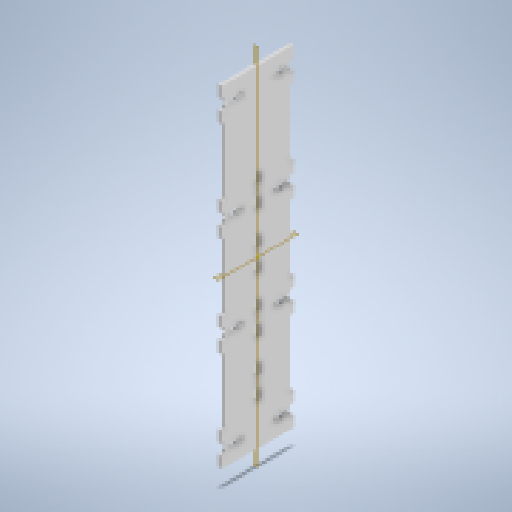
# Autodesk Inventor part: Крепление для крепления механизма головы
Saved by Autodesk Inventor 2023.2 (Build 272271030, 271C)
## iProperties
Created: 2024-02-18
Part Number: Крепление для крепления механизма головы
Material: Типовые
Document SubType Name: Modeling
Designer: I9232
Density: 1 g/cm^3
Appearance: Серо-синий
Mass: 21.1298 g
Surface Area: 152.682 cm^2
Volume: 21.1298 cm^3
Author: I9232
Autodesk Inventor part; units mm, degrees
ref_plane "YZ Plane" through (0, 0, 0) normal (1, 0, 0) x (0, 1, 0)
sketch "Эскиз1" plane through (0, 0, 0) normal (1, 0, 0) x (0, 1, 0)
  line L0 (-150, 29.5) -> (150, 29.5)
  line L1 (150, 29.5) -> (150, -29.5)
  line L2 (150, -29.5) -> (-150, -29.5)
  line L3 (-150, -29.5) -> (-150, 29.5)
  line L4 (-150, 29.5) -> (150, -29.5) construction
  line L5 (150, 29.5) -> (-150, -29.5) construction
  point P0 (0, 0)
  dimension "d0" = 300
  dimension "d1" = 59
  constraints: 12 end point, 2 midpoint, 2 parallel, 1 horizontal, 1 perpendicular
  measures "d0" distance of L0.start L0.end
  measures "d1" distance of L0.end L1.end
extrude "Выдавливание1" add sketch "Эскиз1" along normal mid plane 3
sketch "Эскиз2" plane through (0, 0, 0) normal (1, 0, 0) x (0, 1, 0)
  point P0 (0, 0)
sketch "Эскиз4" plane through (1.5, -150, -29.5) normal (0, 0, -1) x (-1, 0, 0)
  line L0 (3, 0) -> (0, 0)
  line L1 (0, 0) -> (0, 10)
  line L2 (0, 10) -> (3, 10)
  line L3 (3, 10) -> (3, 0)
  line L4 (3, 0) -> (3, 300) projected
  line L5 (0, 0) -> (0, 300) projected
  line L6 (3, 20) -> (0, 20)
  line L7 (0, 20) -> (0, 30)
  line L8 (0, 30) -> (3, 30)
  line L9 (3, 30) -> (3, 20)
  line L10 (3, 120) -> (0, 120)
  line L11 (0, 120) -> (0, 110)
  line L12 (0, 110) -> (3, 110)
  line L13 (3, 110) -> (3, 120)
  line L14 (3, 90) -> (3, 100)
  line L15 (3, 100) -> (0, 100)
  line L16 (0, 100) -> (0, 90)
  line L17 (0, 90) -> (3, 90)
  line L18 (3, 150) -> (0, 150) construction
  line L19 (3, 300) -> (0, 300)
  line L20 (0, 300) -> (0, 290)
  line L21 (0, 290) -> (3, 290)
  line L22 (3, 290) -> (3, 300)
  line L23 (3, 280) -> (0, 280)
  line L24 (0, 280) -> (0, 270)
  line L25 (0, 270) -> (3, 270)
  line L26 (3, 270) -> (3, 280)
  line L27 (3, 180) -> (0, 180)
  line L28 (0, 180) -> (0, 190)
  line L29 (0, 190) -> (3, 190)
  line L30 (3, 190) -> (3, 180)
  line L31 (3, 210) -> (3, 200)
  line L32 (3, 200) -> (0, 200)
  line L33 (0, 200) -> (0, 210)
  line L34 (0, 210) -> (3, 210)
  point P0 (1.5, 150)
  point P1 (1.5, 120)
  point P2 (1.5, 100)
  point P3 (1.5, 180)
  point P4 (1.5, 200)
  point P5 (0, 200)
  point P6 (0, 180)
  point P7 (0, 120)
  point P8 (0, 100)
  dimension "d14" = 10
  dimension "d18" = 20
  dimension "d23" = 30
  dimension "d26" = 20
  constraints: 66 end point, 16 symmetric about line, 4 parallel, 3 midpoint, 2 horizontal, 2 perpendicular, 2 point on line, 2 vertical, 1 collinear, 17 other
  measures "d14" distance of L0.end L1.end
  measures "d18" distance of L1.end L7.end
  measures "d23" distance of point (1.5, 120) point (1.5, 150)
  measures "d26" distance of L10.start L14.end
extrude "Выдавливание2" add sketch "Эскиз4" along normal blind 3 contours L0 L1 L2 L3 | L6 L5 L8 L4 | L17 L5 L15 L4 | L12 L5 L10 L4 | L27 L5 L29 L4 | L32 L5 L34 L4 | L25 L5 L23 L4 | L21 L5 L19 L4
sketch "Эскиз5" plane through (1.5, -150, 29.5) normal (0, 0, 1) x (1, 0, 0)
  line L0 (0, 30) -> (0, 20)
  line L1 (0, 20) -> (-3, 20)
  line L2 (-3, 20) -> (-3, 30)
  line L3 (-3, 30) -> (0, 30)
  line L4 (-3, 10) -> (0, 10)
  line L5 (0, 10) -> (0, 0)
  line L6 (0, 0) -> (-3, 0)
  line L7 (-3, 0) -> (-3, 10)
  line L8 (-3, 90) -> (-3, 100)
  line L9 (-3, 100) -> (0, 100)
  line L10 (0, 100) -> (0, 90)
  line L11 (0, 90) -> (-3, 90)
  line L12 (-3, 110) -> (-3, 120)
  line L13 (-3, 120) -> (0, 120)
  line L14 (0, 120) -> (0, 110)
  line L15 (0, 110) -> (-3, 110)
  line L16 (-3, 180) -> (-3, 190)
  line L17 (-3, 190) -> (0, 190)
  line L18 (0, 190) -> (0, 180)
  line L19 (0, 180) -> (-3, 180)
  line L20 (-3, 200) -> (-3, 210)
  line L21 (-3, 210) -> (0, 210)
  line L22 (0, 210) -> (0, 200)
  line L23 (0, 200) -> (-3, 200)
  line L24 (0, 280) -> (0, 270)
  line L25 (0, 270) -> (-3, 270)
  line L26 (-3, 270) -> (-3, 280)
  line L27 (-3, 280) -> (0, 280)
  line L28 (0, 300) -> (0, 290)
  line L29 (0, 290) -> (-3, 290)
  line L30 (-3, 290) -> (-3, 300)
  line L31 (-3, 300) -> (0, 300)
  point P0 (-1.5, 150)
  constraints: 64 end point
extrude "Выдавливание3" add sketch "Эскиз5" along normal blind 3
sketch "Эскиз6" plane through (1.5, 0, 0) normal (1, 0, 0) x (0, 0, -1)
  line L0 (29.5, -130) -> (29.5, -140) projected
  line L1 (13.9, -136.5) -> (13.9, -133.5)
  line L2 (29.5, -133.5) -> (29.5, -136.5)
  line L3 (21.4, -138.05) -> (18.9, -138.05)
  line L4 (18.9, -131.95) -> (21.4, -131.95)
  line L5 (29.5, -136.5) -> (21.4, -136.5)
  line L6 (18.9, -136.5) -> (13.9, -136.5)
  line L7 (21.4, -131.95) -> (21.4, -133.5)
  line L8 (21.4, -136.5) -> (21.4, -138.05)
  line L9 (18.9, -138.05) -> (18.9, -136.5)
  line L10 (18.9, -133.5) -> (18.9, -131.95)
  line L11 (13.9, -133.5) -> (18.9, -133.5)
  line L12 (21.4, -133.5) -> (29.5, -133.5)
  line L13 (21.4, -138.05) -> (18.9, -131.95) construction
  line L14 (18.9, -138.05) -> (21.4, -131.95) construction
  line L15 (13.9, -46.51) -> (13.9, -43.51)
  line L16 (29.5, -43.5) -> (29.5, -46.5)
  line L17 (21.4, -48.06) -> (18.9, -48.06)
  line L18 (18.9, -41.96) -> (21.4, -41.96)
  line L19 (29.5, -46.5) -> (21.4, -46.5)
  line L20 (18.9, -46.51) -> (13.9, -46.51)
  line L21 (21.4, -41.96) -> (21.4, -43.5)
  line L22 (21.4, -46.5) -> (21.4, -48.06)
  line L23 (18.9, -48.06) -> (18.9, -46.51)
  line L24 (18.9, -43.51) -> (18.9, -41.96)
  line L25 (13.9, -43.51) -> (18.9, -43.51)
  line L26 (21.4, -43.5) -> (29.5, -43.5)
  line L27 (21.4, -48.06) -> (18.9, -41.96) construction
  line L28 (18.9, -48.06) -> (21.4, -41.96) construction
  line L29 (29.5, -50) -> (29.5, -40) projected
  line L30 (0, -102.6029) -> (0, -84.657) construction
  line L31 (-13.9, -136.5) -> (-13.9, -133.5)
  line L32 (-21.4, -138.05) -> (-18.9, -138.05)
  line L33 (-18.9, -131.95) -> (-21.4, -131.95)
  line L34 (-29.5, -136.5) -> (-21.4, -136.5)
  line L35 (-18.9, -136.5) -> (-13.9, -136.5)
  line L36 (-21.4, -131.95) -> (-21.4, -133.5)
  line L37 (-21.4, -136.5) -> (-21.4, -138.05)
  line L38 (-18.9, -138.05) -> (-18.9, -136.5)
  line L39 (-18.9, -133.5) -> (-18.9, -131.95)
  line L40 (-13.9, -133.5) -> (-18.9, -133.5)
  line L41 (-21.4, -133.5) -> (-29.5, -133.5)
  line L42 (-21.4, -138.05) -> (-18.9, -131.95) construction
  line L43 (-18.9, -138.05) -> (-21.4, -131.95) construction
  line L44 (-18.9, -41.96) -> (-21.4, -41.96)
  line L45 (-18.9, -48.06) -> (-21.4, -41.96) construction
  line L46 (-21.4, -48.06) -> (-18.9, -48.06)
  line L47 (-21.4, -48.06) -> (-18.9, -41.96) construction
  line L48 (-21.4, -41.96) -> (-21.4, -43.5)
  line L49 (-21.4, -46.5) -> (-21.4, -48.06)
  line L50 (-29.5, -43.5) -> (-29.5, -46.5)
  line L51 (-21.4, -43.5) -> (-29.5, -43.5)
  line L52 (-29.5, -46.5) -> (-21.4, -46.5)
  line L53 (-18.9, -43.51) -> (-18.9, -41.96)
  line L54 (-18.9, -48.06) -> (-18.9, -46.51)
  line L55 (-18.9, -46.51) -> (-13.9, -46.51)
  line L56 (-13.9, -43.51) -> (-18.9, -43.51)
  line L57 (-13.9, -46.51) -> (-13.9, -43.51)
  line L58 (7.1408, 0) -> (-5.4038, 0) construction
  line L59 (13.9, 136.5) -> (13.9, 133.5)
  line L60 (29.5, 133.5) -> (29.5, 136.5)
  line L61 (21.4, 138.05) -> (18.9, 138.05)
  line L62 (18.9, 131.95) -> (21.4, 131.95)
  line L63 (29.5, 136.5) -> (21.4, 136.5)
  line L64 (18.9, 136.5) -> (13.9, 136.5)
  line L65 (21.4, 131.95) -> (21.4, 133.5)
  line L66 (21.4, 136.5) -> (21.4, 138.05)
  line L67 (18.9, 138.05) -> (18.9, 136.5)
  line L68 (18.9, 133.5) -> (18.9, 131.95)
  line L69 (13.9, 133.5) -> (18.9, 133.5)
  line L70 (21.4, 133.5) -> (29.5, 133.5)
  line L71 (21.4, 138.05) -> (18.9, 131.95) construction
  line L72 (18.9, 138.05) -> (21.4, 131.95) construction
  line L73 (18.9, 41.96) -> (21.4, 41.96)
  line L74 (18.9, 48.06) -> (21.4, 41.96) construction
  line L75 (21.4, 48.06) -> (18.9, 48.06)
  line L76 (21.4, 48.06) -> (18.9, 41.96) construction
  line L77 (21.4, 41.96) -> (21.4, 43.5)
  line L78 (21.4, 46.5) -> (21.4, 48.06)
  line L79 (29.5, 43.5) -> (29.5, 46.5)
  line L80 (21.4, 43.5) -> (29.5, 43.5)
  line L81 (29.5, 46.5) -> (21.4, 46.5)
  line L82 (18.9, 43.51) -> (18.9, 41.96)
  line L83 (18.9, 48.06) -> (18.9, 46.51)
  line L84 (18.9, 46.51) -> (13.9, 46.51)
  line L85 (13.9, 43.51) -> (18.9, 43.51)
  line L86 (13.9, 46.51) -> (13.9, 43.51)
  line L87 (0, 102.6029) -> (0, 84.657) construction
  line L88 (-21.4, 131.95) -> (-21.4, 133.5)
  line L89 (-21.4, 138.05) -> (-18.9, 138.05)
  line L90 (-21.4, 138.05) -> (-18.9, 131.95) construction
  line L91 (-18.9, 138.05) -> (-18.9, 136.5)
  line L92 (-18.9, 131.95) -> (-21.4, 131.95)
  line L93 (-13.9, 133.5) -> (-18.9, 133.5)
  line L94 (-13.9, 136.5) -> (-13.9, 133.5)
  line L95 (-18.9, 136.5) -> (-13.9, 136.5)
  line L96 (-18.9, 138.05) -> (-21.4, 131.95) construction
  line L97 (-18.9, 46.51) -> (-13.9, 46.51)
  line L98 (-13.9, 43.51) -> (-18.9, 43.51)
  line L99 (-13.9, 46.51) -> (-13.9, 43.51)
  line L100 (-18.9, 133.5) -> (-18.9, 131.95)
  line L101 (-21.4, 136.5) -> (-21.4, 138.05)
  line L102 (-21.4, 133.5) -> (-29.5, 133.5)
  line L103 (-29.5, 136.5) -> (-21.4, 136.5)
  line L104 (-18.9, 41.96) -> (-21.4, 41.96)
  line L105 (-18.9, 48.06) -> (-18.9, 46.51)
  line L106 (-21.4, 48.06) -> (-18.9, 48.06)
  line L107 (-21.4, 46.5) -> (-21.4, 48.06)
  line L108 (-18.9, 43.51) -> (-18.9, 41.96)
  line L109 (-18.9, 48.06) -> (-21.4, 41.96) construction
  line L110 (-21.4, 48.06) -> (-18.9, 41.96) construction
  line L111 (-21.4, 41.96) -> (-21.4, 43.5)
  line L112 (-29.5, 46.5) -> (-21.4, 46.5)
  line L113 (-21.4, 43.5) -> (-29.5, 43.5)
  line L114 (-29.5, 129.75) -> (-29.5, 139.75)
  line L115 (-29.5, 43.5) -> (-29.5, 46.5)
  line L116 (-29.5, -136.5) -> (-29.5, -133.5)
  line L117 (-29.5, -140) -> (-29.5, -130) projected
  point P0 (0, 0)
  point P1 (29.5, -135)
  point P2 (21.4, -47.28)
  point P3 (29.5, -45)
  point P4 (-21.4, -47.28)
  point P5 (29.5, 135)
  point P6 (21.4, 47.28)
  point P7 (29.5, 45)
  point P8 (-21.4, 47.28)
  point P9 (29.5, -133.5)
  dimension "d36" = 3
  dimension "d40" = 2.5
  dimension "d42" = 8.1
  dimension "d43" = 8.1
  dimension "d44" = 5
  dimension "d45" = 3
  dimension "d46" = 3
  dimension "d48" = 2.5
  dimension "d51" = 8.1
  dimension "d52" = 5
  dimension "d53" = 3
  dimension "d54" = 8.1
  dimension "d58" = 6.1
  dimension "d59" = 6.1
  constraints: 230 end point, 79 symmetric about line, 20 parallel, 8 perpendicular, 7 horizontal, 5 midpoint, 4 equal length, 2 point on line, 1 collinear, 1 vertical
  measures "d36" distance of L1.start L1.end
  measures "d40" distance of L3.start L3.end
  measures "d42" distance between parallel lines of L0 L8
  measures "d43" distance between parallel lines of L2 L7
  measures "d44" distance of L6.start L1.start
  measures "d45" distance between parallel lines of L12 L5
  measures "d46" distance of L20.end L25.start
  measures "d48" distance of L17.start L28.start
  measures "d51" distance between parallel lines of L16 L21
  measures "d52" distance of L23.end L20.end
  measures "d53" distance between parallel lines of L26 L19
  measures "d54" distance from line of point (21.4, -47.28) L16
  measures "d58" distance between parallel lines of L4 L3
  measures "d59" distance between parallel lines of L18 L17
extrude "Выдавливание4" cut sketch "Эскиз6" against normal blind 3
sketch "Эскиз7" plane through (-1.5, 0, 0) normal (-1, 0, 0) x (0, 0, 1)
  line L0 (2, 57.2151) -> (2, 67.2151) projected
  line L1 (-2, 57.2151) -> (2, 57.2151) projected
  line L2 (-2, 67.2151) -> (-2, 57.2151) projected
  line L3 (2, 67.2151) -> (-2, 67.2151) projected
  line L4 (2, 47.2151) -> (-2, 47.2151) projected
  line L5 (2, 37.2151) -> (2, 47.2151) projected
  line L6 (-2, 47.2151) -> (-2, 37.2151) projected
  line L7 (-2, 37.2151) -> (2, 37.2151) projected
  line L8 (-2, -12.7849) -> (2, -12.7849) projected
  line L9 (2, -12.7849) -> (2, -2.7849) projected
  line L10 (-2, -2.7849) -> (-2, -12.7849) projected
  line L11 (2, -2.7849) -> (-2, -2.7849) projected
  line L12 (-2, 7.2151) -> (2, 7.2151) projected
  line L13 (2, 7.2151) -> (2, 17.2151) projected
  line L14 (-2, 17.2151) -> (-2, 7.2151) projected
  line L15 (2, 17.2151) -> (-2, 17.2151) projected
  line L16 (-2, -62.7849) -> (2, -62.7849) projected
  line L17 (2, -62.7849) -> (2, -52.7849) projected
  line L18 (-2, -52.7849) -> (-2, -62.7849) projected
  line L19 (2, -52.7849) -> (-2, -52.7849) projected
  line L20 (2, -32.7849) -> (-2, -32.7849) projected
  line L21 (2, -42.7849) -> (2, -32.7849) projected
  line L22 (-2, -32.7849) -> (-2, -42.7849) projected
  line L23 (-2, -42.7849) -> (2, -42.7849) projected
  line L24 (-2, -112.7849) -> (2, -112.7849) projected
  line L25 (-2, -102.7849) -> (-2, -112.7849) projected
  line L26 (2, -112.7849) -> (2, -102.7849) projected
  line L27 (2, -102.7849) -> (-2, -102.7849) projected
  line L28 (-2, -92.7849) -> (2, -92.7849) projected
  line L29 (-2, -82.7849) -> (-2, -92.7849) projected
  line L30 (2, -92.7849) -> (2, -82.7849) projected
  line L31 (2, -82.7849) -> (-2, -82.7849) projected
  point P0 (0, 0)
sketch "Эскиз8" plane through (-1.5, 0, 0) normal (-1, 0, 0) x (0, 0, 1)
  circle A0 centre (0, 52.2151) radius 1.5
  circle A1 centre (0, -97.7849) radius 1.5
  circle A2 centre (0, -47.7849) radius 1.5
  circle A3 centre (0, 2.2151) radius 1.5
  line L0 (-2, 57.2151) -> (2, 57.2151) projected
  line L1 (2, 47.2151) -> (-2, 47.2151) projected
  line L2 (2, -2.7849) -> (-2, -2.7849) projected
  line L3 (-2, 7.2151) -> (2, 7.2151) projected
  line L4 (-2, -42.7849) -> (2, -42.7849) projected
  line L5 (2, -52.7849) -> (-2, -52.7849) projected
  line L6 (-2, -92.7849) -> (2, -92.7849) projected
  line L7 (2, -102.7849) -> (-2, -102.7849) projected
  line L8 (0, -102.7849) -> (0, -92.7849) construction
  line L9 (0, -52.7849) -> (0, -42.7849) construction
  line L10 (0, -2.7849) -> (0, 7.2151) construction
  line L11 (0, 47.2151) -> (0, 57.2151) construction
  point P0 (0, 0)
  point P1 (0, 2.2151)
  point P2 (0, -47.7849)
  point P3 (0, -97.7849)
  point P4 (0, 52.2151)
  dimension "d60" = 3
  constraints: 12 midpoint, 8 end point, 4 centre point, 4 coincident, 3 equal radius
  measures "d60" diameter of A0
extrude "Выдавливание5" cut sketch "Эскиз7" against normal up to surface (3 mm away)
extrude "Выдавливание6" cut sketch "Эскиз8" against normal up to surface (3 mm away)
sketch "Эскиз9" plane through (-1.5, 0, 0) normal (-1, 0, 0) x (0, 0, 1)
  line L0 (25, 81.2151) -> (20, 81.2151) projected
  line L1 (20, 81.2151) -> (20, 77.2151) projected
  line L2 (20, 77.2151) -> (25, 77.2151) projected
  line L3 (25, 77.2151) -> (25, 81.2151) projected
  line L4 (10, 81.2151) -> (5, 81.2151) projected
  line L5 (5, 81.2151) -> (5, 77.2151) projected
  line L6 (5, 77.2151) -> (10, 77.2151) projected
  line L7 (10, 77.2151) -> (10, 81.2151) projected
  line L8 (-5, 81.2151) -> (-10, 81.2151) projected
  line L9 (-10, 81.2151) -> (-10, 77.2151) projected
  line L10 (-10, 77.2151) -> (-5, 77.2151) projected
  line L11 (-5, 77.2151) -> (-5, 81.2151) projected
  line L12 (-20, 81.2151) -> (-25, 81.2151) projected
  line L13 (-25, 81.2151) -> (-25, 77.2151) projected
  line L14 (-25, 77.2151) -> (-20, 77.2151) projected
  line L15 (-20, 77.2151) -> (-20, 81.2151) projected
  point P0 (0, 0)
extrude "Выдавливание7" cut sketch "Эскиз9" against normal up to surface (3 mm away)
sketch "Эскиз10" plane through (-1.5, 0, 0) normal (-1, 0, 0) x (0, 0, 1)
  line L0 (20, 81.2151) -> (20, 77.2151) projected
  line L1 (10, 77.2151) -> (10, 81.2151) projected
  line L2 (-10, 81.2151) -> (-10, 77.2151) projected
  line L3 (-20, 77.2151) -> (-20, 81.2151) projected
  line L4 (20, 77.2151) -> (20, 81.2151) projected
  line L5 (20, 79.2151) -> (10, 79.2151) construction
  line L6 (10, 81.2151) -> (10, 77.2151) projected
  line L7 (-10, 77.2151) -> (-10, 81.2151) projected
  line L8 (-10, 79.2151) -> (-20, 79.2151) construction
  line L9 (-20, 81.2151) -> (-20, 77.2151) projected
  circle A0 centre (15, 79.2151) radius 1.5
  circle A1 centre (-15, 79.2151) radius 1.5
  point P0 (0, 0)
  point P1 (15, 79.2151)
  point P2 (-15, 79.2151)
  dimension "d67" = 3
  constraints: 6 midpoint, 4 end point, 2 centre point, 2 coincident, 1 equal radius
  measures "d67" diameter of A0
extrude "Выдавливание8" cut sketch "Эскиз10" against normal up to surface (3 mm away)
